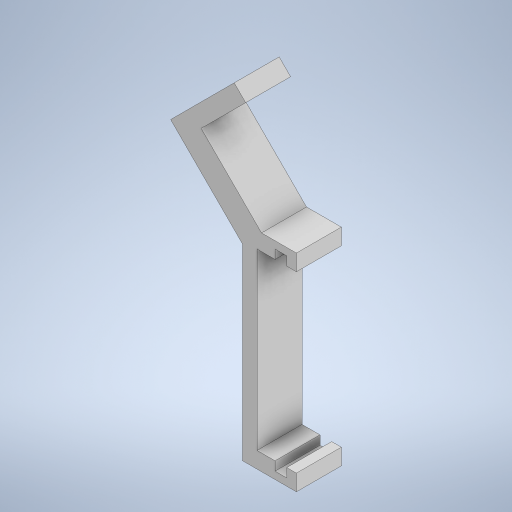
# Autodesk Inventor part: ultrasonic-sensor-direct-mount
Saved by Autodesk Inventor 2023 (Build 270158000, 158)
## iProperties
Created: 2023-02-22
Part Number: ultrasonic-sensor-direct-mount
Material: Generisch
Document SubType Name: Modeling
Designer: tommi
Density: 1 g/cm^3
Appearance: Vorgabe
Author: tommi
Autodesk Inventor part; units mm, degrees
ref_plane "YZ Plane" through (0, 0, 0) normal (1, 0, 0) x (0, 1, 0)
ref_plane "XZ Plane" through (0, 0, 0) normal (0, 1, 0) x (-1, 0, 0)
ref_plane "XY Plane" through (0, 0, 0) normal (0, 0, 1) x (1, 0, 0)
sketch "Skizze1" plane through (0, 0, 0) normal (0, 0, 1) x (1, 0, 0)
  line L0 (-3, 11.5) -> (3, 11.5)
  line L1 (3, 11.5) -> (3, -11.5)
  line L2 (3, -11.5) -> (-3, -11.5)
  line L3 (-3, -11.5) -> (-3, 9.3787)
  line L4 (-3, 11.5) -> (3, -11.5) construction
  line L5 (3, 11.5) -> (-3, -11.5) construction
  line L6 (-3, 0) -> (3, 0)
  line L7 (1.925, 10.6961) -> (1.925, 9.7)
  line L8 (0.625, 10.6961) -> (0.625, 9.7)
  line L9 (-1.375, 9.7) -> (-1.375, 0)
  line L10 (0.625, 10.6961) -> (1.925, 10.6961)
  line L11 (-1.375, 9.7) -> (0.625, 9.7)
  line L12 (1.925, 9.7) -> (3, 9.7)
  line L13 (-3, 0) -> (3, 0)
  line L14 (0.625, -10.6961) -> (0.625, -9.7)
  line L15 (-1.375, -9.7) -> (-1.375, 0)
  line L16 (0.625, -10.6961) -> (1.925, -10.6961)
  line L17 (-1.375, -9.7) -> (0.625, -9.7)
  line L18 (1.925, -9.7) -> (3, -9.7)
  line L19 (1.925, -9.7) -> (1.925, -10.6961)
  line L20 (-0.8787, 11.5) -> (2.008, 11.5) construction
  line L21 (-3, 11.5) -> (4, 11.5) construction
  line L22 (-3, 11.5) -> (4, 11.5) construction
  line L23 (-3, 11.5) -> (-8.6569, 17.1569)
  line L24 (-3, 11.5) -> (5, 11.5) construction
  line L25 (-9.7158, 16.0944) -> (-4.0624, 10.4411)
  line L26 (-4.0624, 10.4411) -> (-1.9411, 12.5624)
  line L27 (-1.9411, 12.5624) -> (-7.5944, 18.2158)
  line L28 (-7.5944, 18.2158) -> (-9.7158, 16.0944)
  line L29 (-9.7158, 16.0944) -> (-1.9411, 12.5624) construction
  line L30 (-4.0624, 10.4411) -> (-7.5944, 18.2158) construction
  line L31 (-9.7158, 16.0944) -> (-2.6447, 23.1655)
  line L32 (-2.6447, 23.1655) -> (-3.9175, 24.4383)
  line L33 (-3.9175, 24.4383) -> (-10.9886, 17.3672)
  line L34 (-10.9886, 17.3672) -> (-9.7158, 16.0944)
  line L35 (-4.0624, 10.4411) -> (-3, 9.3787)
  line L36 (-1.9411, 12.5624) -> (-0.8787, 11.5)
  point P0 (0, 0)
  point P1 (1.925, 10.1981)
  point P2 (-0.7373, 11.5)
  point P3 (-5.8284, 14.3284)
  point P4 (-3, 9.4787)
  point P5 (-0.8787, 11.5)
  point P6 (-7.5944, 18.2158)
  dimension "d0" = 6
  dimension "d1" = 23
  dimension "d19" = 1.3
  dimension "d20" = 2
  dimension "d26" = 1.8
  dimension "d27" = 1.8
  dimension "d40" = 8
  dimension "d41" = 135
  dimension "d42" = 3
  dimension "d43" = 10
  dimension "d44" = 1.8
  constraints: 74 end point, 9 parallel, 8 perpendicular, 7 midpoint, 7 point on line, 6 symmetric about line, 5 horizontal, 2 vertical, 1 equal length
  measures "d0" distance of L1.end L2.end
  measures "d1" distance of L0.end L1.end
  measures "d19" distance between parallel lines of L7 L8
  measures "d20" distance between parallel lines of L9 L8
  measures "d26" distance between parallel lines of L0 L12
  measures "d27" distance between parallel lines of L20 L11
  measures "d40" distance of L0.start L23.end
  measures "d41" angle of L24 L23
  measures "d42" distance of L26.end L25.end
  measures "d43" distance of L25.start L31.end
  measures "d44" distance of L32.end L31.end
extrude "Extrusion1" add sketch "Skizze1" along normal mid plane 5 contours L23 L26 L36 L0 | L0 L1 L12 L7 L10 L8 L11 L9 L6 L3 L35 L26 L23 | L26 L25 L28 L23 | L23 L28 L27 L26 | L28 L34 L33 L32 L31 | L6 L15 L17 L14 L16 L19 L18 L1 L2 L3
sketch "Skizze2" plane through (-2.6447, 23.1655, 2.5) normal (0.7071, -0.7071, 0) x (-0.7071, -0.7071, 0)
  line L0 (0, 5) -> (7, 5) projected
  line L1 (7, 5) -> (10, 5) projected
  line L2 (10, 0) -> (7, 0) projected
  line L3 (7, 0) -> (0, 0) projected
  line L4 (0, 0) -> (0, 5) projected
  line L5 (7, 0) -> (7, 5) projected
  line L6 (7, 0) -> (0, 0) projected
  line L7 (0, 0) -> (0, 5)
  line L8 (0, 5) -> (4, 5)
  line L9 (4, 5) -> (4, 0)
  line L10 (4, 0) -> (0, 0)
  line L11 (0, 0) -> (4, 5)
  circle A0 centre (2, 2.5) radius 0.8
  line L12 (10, 5) -> (10, 0) projected
  point P0 (14.5104, 2.5)
  point P1 (10, 4.5)
  dimension "d45" = 4
  dimension "d46" = 1.6
  constraints: 10 end point, 2 parallel, 2 perpendicular, 1 centre point, 1 midpoint
  measures "d45" distance of L0.start L8.end
  measures "d46" diameter of A0
extrude "Extrusion2" cut sketch "Skizze2" against normal up to surface (1.8 mm away) contours A0 L11 | L11 A0
